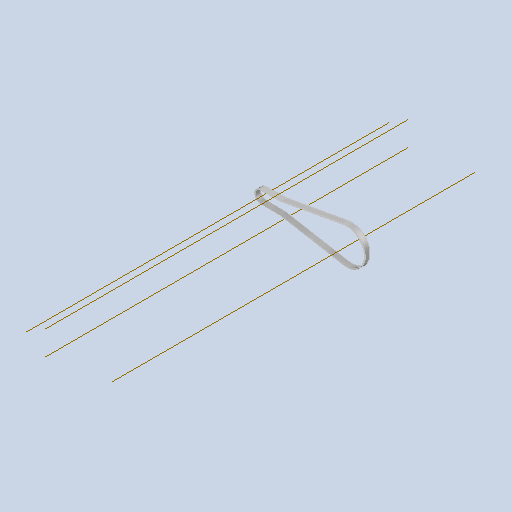
# Autodesk Inventor part: Synchronous Belt
Saved by Autodesk Inventor 2022.2 (Build 262287000, 287)
## iProperties
CustomPartVersion: 1
Created: 2022-01-10
Part Number: Synchronous Belt
Material: Rubber
Document SubType Name: Modeling
Designer: Jochen
Density: 1 g/cm^3
Appearance: Rubber - Black - Version 1.1
Author: Jochen
Autodesk Inventor part; units mm, degrees
ref_plane "YZ Plane" through (0, 0, 0) normal (1, 0, 0) x (0, 1, 0)
ref_plane "XZ Plane" through (0, 0, 0) normal (0, 1, 0) x (-1, 0, 0)
ref_plane "XY Plane" through (0, 0, 0) normal (0, 0, 1) x (1, 0, 0)
sketch "Sketch Path" plane through (0, 0, 0) normal (0, 0, 1) x (1, 0, 0)
  arc A0 (13.481053, 2.67282) -> (13.481053, -6.875851) centre (13.535704, -2.101516) ccw
  arc A1 (28.854646, 2.848799) -> (29.648015, 2.924041) centre (28.799704, 7.648484) ccw
  arc A2 (80.177269, -16.199989) -> (80.177269, 11.996958) centre (82.708759, -2.101516) ccw
  arc A3 (29.648015, -7.127072) -> (28.854646, -7.05183) centre (28.799704, -11.851516) ccw
  line L0 (28.854646, -7.05183) -> (13.481053, -6.875851)
  line L1 (13.481053, 2.67282) -> (28.854646, 2.848799)
  line L2 (29.648015, 2.924041) -> (80.177269, 11.996958)
  line L3 (80.177269, -16.199989) -> (29.648015, -7.127072)
  constraints: 8 end point, 8 point on circle, 4 centre point
ref_plane "Cross Section Plane" through (13.481053, -6.875851, 0) normal (0.9999345, -0.0114461, 0) x (0, 0, 1)
ref_plane "Work Plane2" through (13.535704, -2.101516, 0) normal (-1, 0, 0) x (0, 0, 1)
ref_plane "Work Plane3" through (82.708759, -2.101516, 0) normal (-0.9999382, -0.0111203, 0) x (0, 0, 1)
sketch "Cross Section" plane through (13.481053, -6.875851, 0) normal (0.9999345, -0.0114461, 0) x (0, 0, 1)
  line L0 (-2, 0.3) -> (2, 0.3)
  line L1 (2, 0.3) -> (2, -0.3)
  line L2 (2, -0.3) -> (-2, -0.3)
  line L3 (-2, -0.3) -> (-2, 0.3)
  line L4 (-2, 0) -> (2, 0) construction
  point P0 (0, 0)
  point P1 (0, 0)
  dimension "d0" = 4
  dimension "d4" = 0.3
  dimension "d5" = 0.3
  constraints: 10 end point, 3 midpoint, 2 parallel, 1 coincident, 1 horizontal, 1 perpendicular, 1 other
  measures "d0" distance between parallel lines of L1 L3
  measures "d4" distance between parallel lines of L2 L4
  measures "d5" distance between parallel lines of L4 L0
sweep "Belt" add profiles "Cross Section" path "Sketch Path" path curves L3 A3 L0 A0 L1 A1 L2 A2
equation "\"d0\" = da_B"
equation "\"d4\" = da_a"
equation "\"d5\" = da_a2"
equation "\"da_B\" = 4"
equation "\"da_pb\" = 2.5"
equation "\"da_a\" = 0.3"
equation "\"da_S\" = 1.5"
equation "\"da_Beta\" = 20deg"
equation "\"da_Ht\" = 0.7"
equation "\"da_H\" = 1.3"
equation "\"da_a2\" = 0.3"
body "Solid1"
